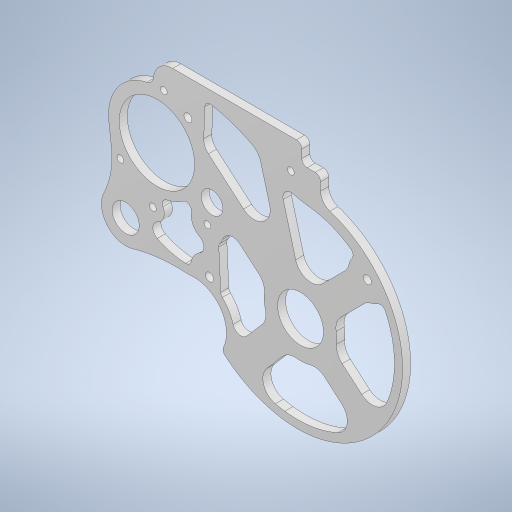
# Autodesk Inventor part: 足内フレーム
Saved by Autodesk Inventor 2023.1 (Build 271208000, 208)
## iProperties
Created: 2022-01-10
Part Number: 足内フレーム
Material: Aluminum 2014-T4
Document SubType Name: Modeling
Designer: acps
Density: 2.8 g/cm^3
Appearance: Satin
Author: acps
Autodesk Inventor part; units mm, degrees
ref_plane "YZ Plane" through (0, 0, 0) normal (1, 0, 0) x (0, 1, 0)
ref_plane "XZ Plane" through (0, 0, 0) normal (0, 1, 0) x (-1, 0, 0)
ref_plane "XY Plane" through (0, 0, 0) normal (0, 0, 1) x (1, 0, 0)
sketch "Sketch9" plane through (0, 0, 0) normal (0, 0, 1) x (1, 0, 0)
  circle A0 centre (46.616, 30) radius 14
  circle A1 centre (67.0906, 21) radius 20.5 construction
  arc A2 (93.8028, -35.6609) -> (110.9454, 40.1044) centre (98.9344, 3) ccw
  arc A3 (71.3782, -23.4684) -> (59.8142, -6.4542) centre (60.4847, -18.4355) ccw
  arc A4 (71.3782, -23.4684) -> (71.8871, -25.8212) centre (73.1938, -24.3072) ccw
  arc A5 (71.8871, -25.8212) -> (93.8028, -35.6609) centre (99.3292, 5.9739) ccw
  circle A6 centre (65.359, 13) radius 3
  circle A7 centre (66.1789, -3.483) radius 4 construction
  circle A8 centre (66.1789, -3.483) radius 3
  circle A9 centre (66.1789, -3.483) radius 1.5
  circle A10 centre (49.1519, 48.073) radius 1.25
  circle A11 centre (45.1, 8.5) radius 1.25
  circle A12 centre (33, 18) radius 1.25
  arc A13 (119.1717, 29.0833) -> (128.6406, 19.1104) centre (124.8574, 25) ccw
  arc A14 (131.5325, 18.2763) -> (128.6406, 19.1104) centre (129.7215, 17.4276) ccw
  arc A15 (119.1717, 29.0833) -> (118.6753, 31.9015) centre (117.5473, 30.25) ccw
  circle A16 centre (67.0906, 21) radius 1.5
  circle A17 centre (67.0906, 21) radius 4.5 construction
  circle A18 centre (49.1519, 48.073) radius 4.25 construction
  arc A19 (42.888, 47.6097) -> (45.3636, 50.3845) centre (42.2376, 50.6816) ccw
  arc A20 (42.888, 47.6097) -> (28.7516, 27.7953) centre (46.616, 30) ccw
  arc A21 (52.4852, 56.8614) -> (45.3636, 50.3845) centre (52.4852, 49.7076) ccw
  arc A22 (118.6753, 31.9015) -> (102.5834, 37.8093) centre (98.9344, 3) ccw
  arc A23 (88.285, 43.2258) -> (102.5834, 37.8093) centre (105.7111, 67.6458) ccw
  arc A24 (88.285, 43.2258) -> (66.7822, 52.3614) centre (56.9182, -0.7301) ccw
  arc A25 (66.7822, 52.3614) -> (64.4184, 50.4721) centre (66.4169, 50.395) ccw
  line L0 (64.4184, 50.4721) -> (63.6467, 30.4665)
  arc A26 (63.6467, 30.4665) -> (65.9495, 28.4127) centre (65.6452, 30.3894) ccw
  arc A27 (72.0057, 15.3351) -> (65.9495, 28.4127) centre (67.0906, 21) ccw
  arc A28 (62.3527, 39.5241) -> (63.2626, 46.965) centre (58.1571, 43.8132) ccw construction
  arc A29 (72.0057, 15.3351) -> (71.327, 13.6183) centre (73.3164, 13.8244) ccw
  arc A30 (70.0506, 9.2598) -> (71.327, 13.6183) centre (65.359, 13) ccw
  arc A31 (63.4085, 27.3516) -> (62.8815, 34.943) centre (46.616, 30) ccw construction
  arc A32 (70.0506, 9.2598) -> (69.6169, 7.9138) centre (71.6145, 8.0131) ccw
  line L1 (69.6169, 7.9138) -> (70.3257, -6.3345)
  arc A33 (70.3257, -6.3345) -> (70.9304, -7.6704) centre (72.3232, -6.2351) ccw
  arc A34 (74.8454, -22.768) -> (70.9304, -7.6704) centre (60.4847, -18.4355) ccw
  arc A35 (75.5402, -24.9305) -> (94.1976, -32.687) centre (99.3292, 5.9739) ccw
  arc A36 (74.8454, -22.768) -> (75.5402, -24.9305) centre (76.7601, -23.3457) ccw
  line L2 (65.359, 13) -> (66.1789, -3.483) construction
  arc A37 (94.1976, -32.687) -> (131.5325, 18.2763) centre (98.9344, 3) ccw
  arc A38 (29.8929, 18.5469) -> (56.821, -6.4645) centre (58.2196, 22.0427) ccw
  arc A39 (50.2005, 13.3822) -> (56.3412, 16.0565) centre (46.616, 30) ccw
  arc A40 (59.4537, 14.062) -> (56.3412, 16.0565) centre (57.4853, 14.4161) ccw
  arc A41 (46.8589, 4.6311) -> (48.8551, 10.4905) centre (45.1, 8.5) ccw
  arc A42 (59.4537, 14.062) -> (62.4846, 7.7333) centre (65.359, 13) ccw
  arc A43 (46.7538, -0.7807) -> (57.3342, -3.4835) centre (58.2196, 22.0427) ccw
  arc A44 (62.5868, 2.5251) -> (59.3536, -1.9287) centre (66.1789, -3.483) ccw
  arc A45 (57.3342, -3.4835) -> (59.3536, -1.9287) centre (57.4035, -1.4847) ccw
  arc A46 (50.2005, 13.3822) -> (48.8551, 10.4905) centre (50.6222, 11.4271) ccw
  arc A47 (62.5868, 2.5251) -> (62.4846, 7.7333) centre (61.0474, 5.1) ccw
  arc A48 (46.8589, 4.6311) -> (46.7538, -0.7807) centre (48.1006, 1.9001) ccw
  circle A49 centre (33, 18) radius 3 construction
  line L3 (29.8929, 18.5469) -> (28.7516, 27.7953)
  circle A50 centre (124.8574, 25) radius 3
  circle A51 centre (124.8574, 25) radius 1.5
  circle A52 centre (100, 0) radius 6.025 construction
  circle A53 centre (100, 0) radius 30 construction
  circle A54 centre (100, 0) radius 8.525
  circle A55 centre (100, 0) radius 13.525
  circle A56 centre (58.1571, 43.8132) radius 3
  circle A57 centre (58.1571, 43.8132) radius 1.5
  arc A58 (116.4268, 23.6124) -> (118.0268, 26.5308) centre (112.172, 27.8429) ccw
  line L4 (116.4268, 23.6124) -> (108.2597, 15.3984)
  arc A59 (126.4272, 18.1783) -> (123.5181, 16.5616) centre (127.7728, 12.3311) ccw
  arc A60 (114.9197, 7.9139) -> (113.2822, 2.5515) centre (119.1744, 3.6834) ccw
  line L5 (114.9197, 7.9139) -> (123.5181, 16.5616)
  line L6 (100, 0) -> (74.542, 21.8523) construction
  arc A61 (91.0161, 14.3009) -> (96.4839, 13.06) centre (94.924, 18.8536) ccw
  arc A62 (86.558, 1.4963) -> (84.5028, 6.7129) centre (80.5949, 2.1601) ccw
  line L7 (77.423, 12.7899) -> (84.5028, 6.7129)
  line L8 (91.0161, 14.3009) -> (65.753, 35.9858)
  arc A63 (77.423, 12.7899) -> (71.0342, 11.0528) centre (74.8177, 9.7547) ccw
  arc A64 (64.0134, 39.9725) -> (65.753, 35.9858) centre (69.0097, 39.7797) ccw
  arc A65 (108.9839, -14.3009) -> (103.5161, -13.06) centre (105.076, -18.8536) ccw
  arc A66 (113.442, -1.4963) -> (115.4972, -6.7129) centre (119.4051, -2.1601) ccw
  line L9 (100, 0) -> (122.764, -19.5398) construction
  line L10 (108.9839, -14.3009) -> (115.3122, -19.7328)
  line L11 (115.4972, -6.7129) -> (122.7736, -12.9587)
  arc A67 (113.8982, -29.7427) -> (115.3122, -19.7328) centre (111.4042, -24.2856) ccw
  arc A68 (122.7736, -12.9587) -> (132.231, -10.6871) centre (126.6816, -8.4059) ccw
  arc A69 (85.6991, -8.9839) -> (86.94, -3.5161) centre (81.1464, -5.076) ccw
  arc A70 (98.5037, -13.442) -> (93.2871, -15.4972) centre (97.8399, -19.4051) ccw
  line L12 (85.6991, -8.9839) -> (80.0896, -15.5191)
  line L13 (87.4521, -22.2951) -> (93.2871, -15.4972)
  arc A71 (74.9251, -14.3768) -> (80.0896, -15.5191) centre (77.8132, -13.5651) ccw
  arc A72 (87.4521, -22.2951) -> (90.6732, -32.0534) centre (92.0049, -26.203) ccw
  circle A73 centre (67.0906, 21) radius 4.025
  arc A74 (78.8207, 24.7689) -> (88.5197, 30.8912) centre (82.7286, 29.3217) ccw
  arc A75 (85.1671, 43.2617) -> (82.1833, 46.995) centre (79.376, 41.6922) ccw
  arc A76 (97.3091, 38.8464) -> (93.5734, 35.1817) centre (96.4689, 35.9664) ccw
  line L14 (85.1671, 43.2617) -> (88.5197, 30.8912)
  line L15 (93.5734, 35.1817) -> (98.2138, 18.0594)
  circle A77 centre (35, 0) radius 5.025
  circle A78 centre (35, 0) radius 9.025
  arc A79 (56.821, -6.4645) -> (37.4687, -8.6808) centre (53.881, -66.3925) ccw
  arc A80 (56.821, -6.4645) -> (59.8142, -6.4542) centre (58.2196, 22.0427) ccw
  line L16 (52.4852, 56.8614) -> (98.4852, 56.8614)
  arc A81 (100.4852, 54.8614) -> (98.4852, 56.8614) centre (98.4852, 54.8614) ccw
  line L17 (100.4852, 54.8614) -> (100.4852, 51.8614)
  arc A82 (100.4852, 51.8614) -> (102.4852, 49.8614) centre (102.4852, 51.8614) ccw
  line L18 (102.4852, 49.8614) -> (105.4852, 49.8614)
  arc A83 (107.4852, 47.8614) -> (105.4852, 49.8614) centre (105.4852, 47.8614) ccw
  line L19 (107.4852, 47.8614) -> (107.4852, 44.8614)
  arc A84 (107.4852, 44.8614) -> (110.9454, 40.1044) centre (112.4852, 44.8614) ccw
  line L20 (100, 0) -> (124.8574, 25) construction
  line L21 (100, 0) -> (88.285, 43.2258) construction
  arc A85 (98.2138, 18.0594) -> (108.2597, 15.3984) centre (104.0049, 19.6289) ccw
  line L22 (69.6707, 28.6693) -> (73.6138, 25.2847) construction
  line L23 (100, 0) -> (77.4284, -26.2961) construction
  circle A86 centre (65.359, 13) radius 1.25
  arc A87 (26.8733, 3.9253) -> (29.6336, 20.6479) centre (-0.1405, 16.9734) ccw
  line L24 (102.4852, 51.8614) -> (91.7278, 41.104) construction
  circle A88 centre (96.3994, 45.7756) radius 1.25
  point P0 (0, 0)
  point P1 (108.4418, 41.9202)
  point P2 (103.9852, 49.8614)
  point P3 (87.271, 10.9261)
  point P4 (58.3178, -6.4986)
  point P5 (40.0247, 0.0526)
  point P6 (35.3136, 5.0152)
  point P7 (101.071, 50.4472)
  dimension "d572" = 2
  dimension "d573" = 42
  dimension "d574" = 74
  dimension "d575" = 118
  dimension "d576" = 6
  dimension "d577" = 8
  dimension "d578" = 6
  dimension "d579" = 3
  dimension "d580" = 2.5
  dimension "d581" = 2.5
  dimension "d582" = 8.5
  dimension "d583" = 45.1
  dimension "d584" = 2.5
  dimension "d585" = 18
  dimension "d586" = 33
  dimension "d587" = 2
  dimension "d588" = 2
  dimension "d589" = 3
  dimension "d590" = 3
  dimension "d591" = 3
  dimension "d592" = 4
  dimension "d593" = 2
  dimension "d594" = 2
  dimension "d595" = 3
  dimension "d596" = 2
  dimension "d597" = 3
  dimension "d598" = 3
  dimension "d599" = 2
  dimension "d600" = 2
  dimension "d601" = 3
  dimension "d602" = 2
  dimension "d603" = 3
  dimension "d604" = 12
  dimension "d605" = 3
  dimension "d606" = 2
  dimension "d607" = 3
  dimension "d608" = 3
  dimension "d609" = 3
  dimension "d610" = 3
  dimension "d611" = 2
  dimension "d612" = 3
  dimension "d613" = 3
  dimension "d614" = 2
  dimension "d615" = 6
  dimension "d616" = 4
  dimension "d617" = 17.05
  dimension "d618" = 5
  dimension "d619" = 3
  dimension "d620" = 6
  dimension "d621" = 6
  dimension "d622" = 6
  dimension "d623" = 6
  dimension "d624" = 6
  dimension "d625" = 10
  dimension "d626" = 5
  dimension "d627" = 4
  dimension "d628" = 5
  dimension "d629" = 6
  dimension "d630" = 6
  dimension "d631" = 10
  dimension "d632" = 5
  dimension "d633" = 6
  dimension "d634" = 6
  dimension "d635" = 6
  constraints: 144 point on circle, 87 centre point, 79 tangent, 50 end point, 12 parallel, 11 concentric, 10 coincident, 5 point on line, 2 midpoint, 2 perpendicular, 2 vertical, 1 horizontal, 1 horizontal alignment, 48 other
  measures "d572" radius of A4
  measures "d573" radius of A5
  measures "d576" diameter of A6
  measures "d577" diameter of A7
  measures "d578" diameter of A8
  measures "d579" diameter of A9
  measures "d580" diameter of A10
  measures "d581" diameter of A11
  measures "d582" vertical distance of point (0, 0) A11.centre
  measures "d583" horizontal distance of point (0, 0) A11.centre
  measures "d584" diameter of A12
  measures "d585" vertical distance of point (0, 0) A12.centre
  measures "d586" horizontal distance of point (0, 0) A12.centre
  measures "d587" radius of A14
  measures "d588" radius of A15
  measures "d589" diameter of A16
  measures "d590" radial gap between concentric circles of A16 A17
  measures "d591" radial gap between concentric circles of A10 A18
  measures "d592" radial gap between concentric circles of A22 A2
  measures "d593" radius of A25
  measures "d594" radius of A26
  measures "d595" radial gap between concentric circles of A17 A27
  measures "d596" radius of A29
  measures "d597" radial gap between concentric circles of A6 A30
  measures "d598" radial gap between concentric circles of A0 A31
  measures "d599" radius of A32
  measures "d600" radius of A33
  measures "d601" radial gap between concentric circles of A3 A34
  measures "d602" radius of A36
  measures "d603" radial gap between concentric circles of A2 A37
  measures "d604" radius of A3
  measures "d605" radial gap between concentric circles of A0 A39
  measures "d606" radius of A40
  measures "d607" radial gap between concentric circles of A11 A41
  measures "d608" radial gap between concentric circles of A6 A42
  measures "d609" radial gap between concentric circles of A38 A43
  measures "d610" radial gap between concentric circles of A44 A7
  measures "d611" radius of A46
  measures "d612" radius of A47
  measures "d613" radius of A48
  measures "d614" radius of A45
  measures "d615" diameter of A49
  measures "d616" radial gap between concentric circles of A13 A50
  measures "d617" diameter of A54
  measures "d619" radial gap between concentric circles of A28 A56
  measures "d620" radius of A58
  measures "d621" radius of A59
  measures "d622" radius of A60
  measures "d623" radius of A61
  measures "d624" radius of A62
  measures "d625" distance between parallel lines of L7 L8
  measures "d626" distance between parallel lines of L8 L6
  measures "d627" radius of A63
  measures "d628" radius of A64
  measures "d629" radius of A65
  measures "d630" radius of A66
  measures "d631" distance between parallel lines of L10 L11
  measures "d632" distance between parallel lines of L11 L9
  measures "d633" radius of A67
  measures "d634" radius of A68
  measures "d635" radius of A69
extrude "Extrusion8" add sketch "Sketch9" along normal blind 3 contours A5 A4 A3 A80 A38 A78 L3 A20 A19 A21 L16 A81 L17 A82 L18 A83 L19 A84 A2 | A79 A78 A38 | A78 A38 A77 | A38 A77 A78 | A87 L3 A38 A78 | A6 | A8 | A13 A59 L5 A60 A55 A61 L8 A74 L14 A75 A24 A23 A76 L15 A85 L4 A58 | A37 A67 L10 A65 A55 A66 L11 A68 | A55 | A55 A62 L7 A63 A30 A29 A27 A26 L0 A64 L8 A61 | A35 A36 A34 A71 L12 A69 A55 A70 L13 A72 | A50 | A56
sketch "sesaku" plane through (0, 0, 0) normal (0, 0, -1) x (1, 0, 0)
  circle A0 centre (124.8574, 25) radius 3 projected
  circle A1 centre (65.359, 13) radius 3 projected
  circle A2 centre (58.1571, 43.8132) radius 3 projected
  arc A3 (57.8161, -6.496) -> (38.145, -9.5189) centre (56.9678, -66.49) ccw projected
  arc A4 (57.8161, -6.496) -> (59.8142, -6.4542) centre (58.2196, 22.0427) ccw projected
  arc A5 (71.3782, -23.4684) -> (59.8142, -6.4542) centre (60.4847, -18.4355) ccw projected
  arc A6 (71.3782, -23.4684) -> (71.8871, -25.8212) centre (73.1938, -24.3072) ccw projected
  arc A7 (71.8871, -25.8212) -> (93.8028, -35.6609) centre (99.3292, 5.9739) ccw projected
  arc A8 (93.8028, -35.6609) -> (110.9454, 40.1044) centre (98.9344, 3) ccw projected
  arc A9 (107.4852, 44.8614) -> (110.9454, 40.1044) centre (112.4852, 44.8614) ccw projected
  line L0 (107.4852, 44.8614) -> (107.4852, 47.8614) projected
  arc A10 (107.4852, 47.8614) -> (105.4852, 49.8614) centre (105.4852, 47.8614) ccw projected
  line L1 (105.4852, 49.8614) -> (102.4852, 49.8614) projected
  arc A11 (100.4852, 51.8614) -> (102.4852, 49.8614) centre (102.4852, 51.8614) ccw projected
  line L2 (100.4852, 51.8614) -> (100.4852, 54.8614) projected
  arc A12 (100.4852, 54.8614) -> (98.4852, 56.8614) centre (98.4852, 54.8614) ccw projected
  line L3 (98.4852, 56.8614) -> (52.4852, 56.8614) projected
  arc A13 (52.4852, 56.8614) -> (45.3636, 50.3845) centre (52.4852, 49.7076) ccw projected
  arc A14 (42.888, 47.6097) -> (45.3636, 50.3845) centre (42.2376, 50.6816) ccw projected
  arc A15 (42.888, 47.6097) -> (28.7516, 27.7953) centre (46.616, 30) ccw projected
  line L4 (28.7516, 27.7953) -> (29.584, 21.0499) projected
  arc A16 (25.6574, 3.6354) -> (29.584, 21.0499) centre (-30.2585, 25.3934) ccw projected
  arc A17 (25.6574, 3.6354) -> (38.145, -9.5189) centre (35, 0) ccw projected
  circle A18 centre (35, 0) radius 5.025 projected
  arc A19 (126.4272, 18.1783) -> (128.6406, 19.1104) centre (124.8574, 25) ccw projected
  arc A20 (131.5325, 18.2763) -> (128.6406, 19.1104) centre (129.7215, 17.4276) ccw projected
  arc A21 (132.231, -10.6871) -> (131.5325, 18.2763) centre (98.9344, 3) ccw projected
  arc A22 (122.7736, -12.9587) -> (132.231, -10.6871) centre (126.6816, -8.4059) ccw projected
  line L5 (122.7736, -12.9587) -> (115.4972, -6.7129) projected
  arc A23 (113.442, -1.4963) -> (115.4972, -6.7129) centre (119.4051, -2.1601) ccw projected
  arc A24 (113.442, -1.4963) -> (113.2822, 2.5515) centre (100, 0) ccw projected
  arc A25 (114.9197, 7.9139) -> (113.2822, 2.5515) centre (119.1744, 3.6834) ccw projected
  line L6 (114.9197, 7.9139) -> (123.5181, 16.5616) projected
  arc A26 (126.4272, 18.1783) -> (123.5181, 16.5616) centre (127.7728, 12.3311) ccw projected
  arc A27 (116.4268, 23.6124) -> (118.0268, 26.5308) centre (112.172, 27.8429) ccw projected
  line L7 (116.4268, 23.6124) -> (108.2597, 15.3984) projected
  arc A28 (98.2138, 18.0594) -> (108.2597, 15.3984) centre (104.0049, 19.6289) ccw projected
  line L8 (98.2138, 18.0594) -> (93.5734, 35.1817) projected
  arc A29 (97.3091, 38.8464) -> (93.5734, 35.1817) centre (96.4689, 35.9664) ccw projected
  arc A30 (97.3091, 38.8464) -> (102.5834, 37.8093) centre (105.7111, 67.6458) ccw projected
  arc A31 (118.6753, 31.9015) -> (102.5834, 37.8093) centre (98.9344, 3) ccw projected
  arc A32 (119.1717, 29.0833) -> (118.6753, 31.9015) centre (117.5473, 30.25) ccw projected
  arc A33 (119.1717, 29.0833) -> (118.0268, 26.5308) centre (124.8574, 25) ccw projected
  arc A34 (108.9839, -14.3009) -> (103.5161, -13.06) centre (105.076, -18.8536) ccw projected
  line L9 (108.9839, -14.3009) -> (115.3122, -19.7328) projected
  arc A35 (113.8982, -29.7427) -> (115.3122, -19.7328) centre (111.4042, -24.2856) ccw projected
  arc A36 (94.1976, -32.687) -> (113.8982, -29.7427) centre (98.9344, 3) ccw projected
  arc A37 (90.6732, -32.0534) -> (94.1976, -32.687) centre (99.3292, 5.9739) ccw projected
  arc A38 (87.4521, -22.2951) -> (90.6732, -32.0534) centre (92.0049, -26.203) ccw projected
  line L10 (87.4521, -22.2951) -> (93.2871, -15.4972) projected
  arc A39 (98.5037, -13.442) -> (93.2871, -15.4972) centre (97.8399, -19.4051) ccw projected
  arc A40 (98.5037, -13.442) -> (103.5161, -13.06) centre (100, 0) ccw projected
  arc A41 (85.1671, 43.2617) -> (82.1833, 46.995) centre (79.376, 41.6922) ccw projected
  line L11 (85.1671, 43.2617) -> (88.5197, 30.8912) projected
  arc A42 (78.8207, 24.7689) -> (88.5197, 30.8912) centre (82.7286, 29.3217) ccw projected
  line L12 (78.8207, 24.7689) -> (65.753, 35.9858) projected
  arc A43 (64.0134, 39.9725) -> (65.753, 35.9858) centre (69.0097, 39.7797) ccw projected
  line L13 (64.0134, 39.9725) -> (64.4184, 50.4721) projected
  arc A44 (66.7822, 52.3614) -> (64.4184, 50.4721) centre (66.4169, 50.395) ccw projected
  arc A45 (82.1833, 46.995) -> (66.7822, 52.3614) centre (56.9182, -0.7301) ccw projected
  circle A46 centre (100, 0) radius 8.525 projected
  circle A47 centre (49.1519, 48.073) radius 1.25 projected
  circle A48 centre (67.0906, 21) radius 4.025 projected
  arc A49 (46.8589, 4.6311) -> (48.8551, 10.4905) centre (45.1, 8.5) ccw projected
  arc A50 (50.2005, 13.3822) -> (48.8551, 10.4905) centre (50.6222, 11.4271) ccw projected
  arc A51 (50.2005, 13.3822) -> (56.3412, 16.0565) centre (46.616, 30) ccw projected
  arc A52 (59.4537, 14.062) -> (56.3412, 16.0565) centre (57.4853, 14.4161) ccw projected
  arc A53 (59.4537, 14.062) -> (62.4846, 7.7333) centre (65.359, 13) ccw projected
  arc A54 (62.5868, 2.5251) -> (62.4846, 7.7333) centre (61.0474, 5.1) ccw projected
  arc A55 (62.5868, 2.5251) -> (59.3536, -1.9287) centre (66.1789, -3.483) ccw projected
  arc A56 (57.3342, -3.4835) -> (59.3536, -1.9287) centre (57.4035, -1.4847) ccw projected
  arc A57 (46.7538, -0.7807) -> (57.3342, -3.4835) centre (58.2196, 22.0427) ccw projected
  arc A58 (46.8589, 4.6311) -> (46.7538, -0.7807) centre (48.1006, 1.9001) ccw projected
  circle A59 centre (33, 18) radius 1.25 projected
  circle A60 centre (45.1, 8.5) radius 1.25 projected
  circle A61 centre (46.616, 30) radius 14 projected
  arc A62 (86.558, 1.4963) -> (86.94, -3.5161) centre (100, 0) ccw projected
  arc A63 (85.6991, -8.9839) -> (86.94, -3.5161) centre (81.1464, -5.076) ccw projected
  line L14 (85.6991, -8.9839) -> (80.0896, -15.5191) projected
  arc A64 (74.9251, -14.3768) -> (80.0896, -15.5191) centre (77.8132, -13.5651) ccw projected
  arc A65 (74.9251, -14.3768) -> (70.9304, -7.6704) centre (60.4847, -18.4355) ccw projected
  arc A66 (70.3257, -6.3345) -> (70.9304, -7.6704) centre (72.3232, -6.2351) ccw projected
  line L15 (70.3257, -6.3345) -> (69.6169, 7.9138) projected
  arc A67 (70.0506, 9.2598) -> (69.6169, 7.9138) centre (71.6145, 8.0131) ccw projected
  arc A68 (70.0506, 9.2598) -> (71.0342, 11.0528) centre (65.359, 13) ccw projected
  arc A69 (77.423, 12.7899) -> (71.0342, 11.0528) centre (74.8177, 9.7547) ccw projected
  line L16 (77.423, 12.7899) -> (84.5028, 6.7129) projected
  arc A70 (86.558, 1.4963) -> (84.5028, 6.7129) centre (80.5949, 2.1601) ccw projected
  circle A71 centre (66.1789, -3.483) radius 1.5 projected
  circle A72 centre (65.359, 13) radius 1.25 projected
  circle A73 centre (58.1571, 43.8132) radius 1.5 projected
  circle A74 centre (124.8574, 25) radius 1.5 projected
  point P0 (0, 0)
body "Solid3"
